Autodesk Inventor part; units mm, degrees
(part 3 of 8)
  line L1096 (-20.811, -20.7427) -> (-20.811, -20.5345) construction
  line L1097 (-20.811, -20.5345) -> (-20.6029, -20.5345) construction
  line L1098 (-20.6029, -20.5345) -> (-20.3947, -20.5345)
  spline S238 degree 2 poles (-20.3947, -20.5345) (-20.2004, -20.5345) (-20.0859, -20.4062) knots 0 0 0 1 1 1
  line L1099 (-20.3947, -20.5345) -> (-20.2004, -20.5345) construction
  line L1100 (-20.2004, -20.5345) -> (-20.0859, -20.4062) construction
  spline S239 degree 2 poles (-20.0859, -20.4062) (-19.9819, -20.2882) (-19.9819, -20.1182) knots 0 0 0 1 1 1
  line L1101 (-20.0859, -20.4062) -> (-19.9819, -20.2882) construction
  line L1102 (-19.9819, -20.2882) -> (-19.9819, -20.1182) construction
  spline S240 degree 2 poles (-19.9819, -20.1182) (-19.9819, -19.9482) (-20.0859, -19.8337) knots 0 0 0 1 1 1
  line L1103 (-19.9819, -20.1182) -> (-19.9819, -19.9482) construction
  line L1104 (-19.9819, -19.9482) -> (-20.0859, -19.8337) construction
  spline S241 degree 2 poles (-20.0859, -19.8337) (-20.2004, -19.7053) (-20.3982, -19.7053) knots 0 0 0 1 1 1
  line L1105 (-20.0859, -19.8337) -> (-20.2004, -19.7053) construction
  line L1106 (-20.2004, -19.7053) -> (-20.3982, -19.7053) construction
  line L1107 (-20.3982, -19.7053) -> (-20.6063, -19.7053)
  spline S242 degree 2 poles (-20.6063, -19.7053) (-20.8873, -19.7053) (-21.1024, -19.8719) knots 0 0 0 1 1 1
  line L1108 (-20.6063, -19.7053) -> (-20.8873, -19.7053) construction
  line L1109 (-20.8873, -19.7053) -> (-21.1024, -19.8719) construction
  spline S243 degree 2 poles (-21.1024, -19.8719) (-21.1649, -19.917) (-21.2308, -19.917) knots 0 0 0 1 1 1
  line L1110 (-21.1024, -19.8719) -> (-21.1649, -19.917) construction
  line L1111 (-21.1649, -19.917) -> (-21.2308, -19.917) construction
  spline S244 degree 2 poles (-21.2308, -19.917) (-21.3141, -19.917) (-21.439, -19.7886) (-21.439, -19.7019) knots 0 0 0 1 2 2 2
  line L1112 (-21.2308, -19.917) -> (-21.3141, -19.917) construction
  line L1113 (-21.3141, -19.917) -> (-21.439, -19.7886) construction
  line L1114 (-21.439, -19.7886) -> (-21.439, -19.7019) construction
  spline S245 degree 2 poles (-21.439, -19.7019) (-21.439, -19.6047) (-21.3522, -19.5388) knots 0 0 0 1 1 1
  line L1115 (-21.439, -19.7019) -> (-21.439, -19.6047) construction
  line L1116 (-21.439, -19.6047) -> (-21.3522, -19.5388) construction
  spline S246 degree 2 poles (-21.3522, -19.5388) (-21.0296, -19.289) (-20.6063, -19.289) knots 0 0 0 1 1 1
  line L1117 (-21.3522, -19.5388) -> (-21.0296, -19.289) construction
  line L1118 (-21.0296, -19.289) -> (-20.6063, -19.289) construction
  line L1119 (-20.6063, -19.289) -> (-20.3982, -19.289)
  spline S247 degree 2 poles (-20.3982, -19.289) (-20.0061, -19.289) (-19.7737, -19.5458) knots 0 0 0 1 1 1
  line L1120 (-20.3982, -19.289) -> (-20.0061, -19.289) construction
  line L1121 (-20.0061, -19.289) -> (-19.7737, -19.5458) construction
  spline S248 degree 2 poles (-19.7737, -19.5458) (-19.5655, -19.7817) (-19.5655, -20.1182) knots 0 0 0 1 1 1
  line L1122 (-19.7737, -19.5458) -> (-19.5655, -19.7817) construction
  line L1123 (-19.5655, -19.7817) -> (-19.5655, -20.1182) construction
  spline S249 degree 2 poles (-19.5655, -20.1182) (-19.5655, -20.5033) (-19.8257, -20.7427) knots 0 0 0 1 1 1
  line L1124 (-19.5655, -20.1182) -> (-19.5655, -20.5033) construction
  line L1125 (-19.5655, -20.5033) -> (-19.8257, -20.7427) construction
  spline S250 degree 2 poles (-19.8257, -20.7427) (-19.5655, -20.9821) (-19.5655, -21.3672) knots 0 0 0 1 1 1
  line L1126 (-19.8257, -20.7427) -> (-19.5655, -20.9821) construction
  line L1127 (-19.5655, -20.9821) -> (-19.5655, -21.3672) construction
  spline S251 degree 2 poles (-19.5655, -21.3672) (-19.5655, -21.7072) (-19.7737, -21.9396) knots 0 0 0 1 1 1
  line L1128 (-19.5655, -21.3672) -> (-19.5655, -21.7072) construction
  line L1129 (-19.5655, -21.7072) -> (-19.7737, -21.9396) construction
  spline S252 degree 2 poles (-19.7737, -21.9396) (-20.0061, -22.1963) (-20.3982, -22.1963) knots 0 0 0 1 1 1
  line L1130 (-19.7737, -21.9396) -> (-20.0061, -22.1963) construction
  line L1131 (-20.0061, -22.1963) -> (-20.3982, -22.1963) construction
  line L1132 (-20.3982, -22.1963) -> (-20.6063, -22.1963)
  spline S253 degree 2 poles (-20.6063, -22.1963) (-21.0296, -22.1963) (-21.3522, -21.9465) knots 0 0 0 1 1 1
  line L1133 (-20.6063, -22.1963) -> (-21.0296, -22.1963) construction
  line L1134 (-21.0296, -22.1963) -> (-21.3522, -21.9465) construction
  spline S254 degree 2 poles (-21.3522, -21.9465) (-21.439, -21.8806) (-21.439, -21.7835) knots 0 0 0 1 1 1
  line L1135 (-21.3522, -21.9465) -> (-21.439, -21.8806) construction
  line L1136 (-21.439, -21.8806) -> (-21.439, -21.7835) construction
  spline S255 degree 2 poles (-21.439, -21.7835) (-21.439, -21.6967) (-21.3141, -21.5684) (-21.2308, -21.5684) knots 0 0 0 1 2 2 2
  line L1137 (-21.439, -21.7835) -> (-21.439, -21.6967) construction
  line L1138 (-21.439, -21.6967) -> (-21.3141, -21.5684) construction
  line L1139 (-21.3141, -21.5684) -> (-21.2308, -21.5684) construction
  spline S256 degree 2 poles (-21.2308, -21.5684) (-21.1649, -21.5684) (-21.1024, -21.6135) knots 0 0 0 1 1 1
  line L1140 (-21.2308, -21.5684) -> (-21.1649, -21.5684) construction
  line L1141 (-21.1649, -21.5684) -> (-21.1024, -21.6135) construction
  spline S257 degree 2 poles (-21.1024, -21.6135) (-20.8873, -21.78) (-20.6063, -21.78) knots 0 0 0 1 1 1
  line L1142 (-21.1024, -21.6135) -> (-20.8873, -21.78) construction
  line L1143 (-20.8873, -21.78) -> (-20.6063, -21.78) construction
  line L1144 (-20.6063, -21.78) -> (-20.3982, -21.78)
  spline S258 degree 2 poles (-20.3982, -21.78) (-20.2004, -21.78) (-20.0859, -21.6482) knots 0 0 0 1 1 1
  line L1145 (-20.3982, -21.78) -> (-20.2004, -21.78) construction
  line L1146 (-20.2004, -21.78) -> (-20.0859, -21.6482) construction
  spline S259 degree 2 poles (-20.0859, -21.6482) (-19.9819, -21.5302) (-19.9819, -21.3602) knots 0 0 0 1 1 1
  line L1147 (-20.0859, -21.6482) -> (-19.9819, -21.5302) construction
  line L1148 (-19.9819, -21.5302) -> (-19.9819, -21.3602) construction
  spline S260 degree 2 poles (-19.9819, -21.3602) (-19.9819, -20.989) (-20.3427, -20.9508) knots 0 0 0 1 1 1
  line L1149 (-19.9819, -21.3602) -> (-19.9819, -20.989) construction
  line L1150 (-19.9819, -20.989) -> (-20.3427, -20.9508) construction
  line L1151 (-20.3427, -20.9508) -> (-20.6029, -20.9508)
  spline S261 degree 2 poles (9.298, -10.1686) (9.0898, -10.1686) (9.0898, -9.9605) knots 0 0 0 1 1 1
  line L1152 (9.298, -10.1686) -> (9.0898, -10.1686) construction
  line L1153 (9.0898, -10.1686) -> (9.0898, -9.9605) construction
  line L1154 (9.0898, -9.9605) -> (9.0898, -8.094)
  spline S262 degree 2 poles (9.0898, -8.094) (9.0898, -7.924) (8.847, -7.6777) (8.677, -7.6777) knots 0 0 0 1 2 2 2
  line L1155 (9.0898, -8.094) -> (9.0898, -7.924) construction
  line L1156 (9.0898, -7.924) -> (8.847, -7.6777) construction
  line L1157 (8.847, -7.6777) -> (8.677, -7.6777) construction
  spline S263 degree 2 poles (7.8478, -9.9605) (7.8478, -10.1686) (7.6397, -10.1686) knots 0 0 0 1 1 1
  line L1158 (7.8478, -9.9605) -> (7.8478, -10.1686) construction
  line L1159 (7.8478, -10.1686) -> (7.6397, -10.1686) construction
  spline S264 degree 2 poles (7.6397, -10.1686) (7.4315, -10.1686) (7.4315, -9.9605) knots 0 0 0 1 1 1
  line L1160 (7.6397, -10.1686) -> (7.4315, -10.1686) construction
  line L1161 (7.4315, -10.1686) -> (7.4315, -9.9605) construction
  line L1162 (7.4315, -9.9605) -> (7.4315, -7.4695)
  spline S265 degree 2 poles (7.4315, -7.4695) (7.4315, -7.2613) (7.6397, -7.2613) knots 0 0 0 1 1 1
  line L1163 (7.4315, -7.4695) -> (7.4315, -7.2613) construction
  line L1164 (7.4315, -7.2613) -> (7.6397, -7.2613) construction
  line L1165 (7.6397, -7.2613) -> (8.677, -7.2613)
  spline S266 degree 2 poles (8.677, -7.2613) (9.0204, -7.2613) (9.5062, -7.747) (9.5062, -8.0905) knots 0 0 0 1 2 2 2
  line L1166 (8.677, -7.2613) -> (9.0204, -7.2613) construction
  line L1167 (9.0204, -7.2613) -> (9.5062, -7.747) construction
  line L1168 (9.5062, -7.747) -> (9.5062, -8.0905) construction
  line L1169 (9.5062, -8.0905) -> (9.5062, -9.9605)
  spline S267 degree 2 poles (9.5062, -9.9605) (9.5062, -10.1686) (9.298, -10.1686) knots 0 0 0 1 1 1
  line L1170 (9.5062, -9.9605) -> (9.5062, -10.1686) construction
  line L1171 (9.5062, -10.1686) -> (9.298, -10.1686) construction
  spline S268 degree 2 poles (5.7697, -9.7523) (5.9397, -9.7523) (6.1825, -9.506) (6.1825, -9.336) knots 0 0 0 1 2 2 2
  line L1172 (5.7697, -9.7523) -> (5.9397, -9.7523) construction
  line L1173 (5.9397, -9.7523) -> (6.1825, -9.506) construction
  line L1174 (6.1825, -9.506) -> (6.1825, -9.336) construction
  spline S269 degree 2 poles (5.3534, -7.6777) (5.1834, -7.6777) (4.9405, -7.924) (4.9405, -8.094) knots 0 0 0 1 2 2 2
  line L1175 (5.3534, -7.6777) -> (5.1834, -7.6777) construction
  line L1176 (5.1834, -7.6777) -> (4.9405, -7.924) construction
  line L1177 (4.9405, -7.924) -> (4.9405, -8.094) construction
  line L1178 (4.9405, -8.094) -> (4.9405, -9.336)
  spline S270 degree 2 poles (4.9405, -9.336) (4.9405, -9.506) (5.1834, -9.7523) (5.3534, -9.7523) knots 0 0 0 1 2 2 2
  line L1179 (4.9405, -9.336) -> (4.9405, -9.506) construction
  line L1180 (4.9405, -9.506) -> (5.1834, -9.7523) construction
  line L1181 (5.1834, -9.7523) -> (5.3534, -9.7523) construction
  line L1182 (5.3534, -9.7523) -> (5.7697, -9.7523)
  line L1183 (5.7697, -10.1686) -> (5.3534, -10.1686)
  spline S271 degree 2 poles (5.3534, -10.1686) (5.0134, -10.1686) (4.5242, -9.6829) (4.5242, -9.3395) knots 0 0 0 1 2 2 2
  line L1184 (5.3534, -10.1686) -> (5.0134, -10.1686) construction
  line L1185 (5.0134, -10.1686) -> (4.5242, -9.6829) construction
  line L1186 (4.5242, -9.6829) -> (4.5242, -9.3395) construction
  line L1187 (4.5242, -9.3395) -> (4.5242, -8.0905)
  spline S272 degree 2 poles (4.5242, -8.0905) (4.5242, -7.747) (5.0134, -7.2613) (5.3534, -7.2613) knots 0 0 0 1 2 2 2
  line L1188 (4.5242, -8.0905) -> (4.5242, -7.747) construction
  line L1189 (4.5242, -7.747) -> (5.0134, -7.2613) construction
  line L1190 (5.0134, -7.2613) -> (5.3534, -7.2613) construction
  line L1191 (5.3534, -7.2613) -> (6.3907, -7.2613)
  spline S273 degree 2 poles (6.3907, -7.2613) (6.5989, -7.2613) (6.5989, -7.4695) knots 0 0 0 1 1 1
  line L1192 (6.3907, -7.2613) -> (6.5989, -7.2613) construction
  line L1193 (6.5989, -7.2613) -> (6.5989, -7.4695) construction
  line L1194 (6.5989, -7.4695) -> (6.5989, -9.3325)
  spline S274 degree 2 poles (6.5989, -9.3325) (6.5989, -9.6448) (6.8903, -9.7697) knots 0 0 0 1 1 1
  line L1195 (6.5989, -9.3325) -> (6.5989, -9.6448) construction
  line L1196 (6.5989, -9.6448) -> (6.8903, -9.7697) construction
  spline S275 degree 2 poles (6.8903, -9.7697) (7.0186, -9.8217) (7.0186, -9.9535) knots 0 0 0 1 1 1
  line L1197 (6.8903, -9.7697) -> (7.0186, -9.8217) construction
  line L1198 (7.0186, -9.8217) -> (7.0186, -9.9535) construction
  spline S276 degree 2 poles (7.0186, -9.9535) (7.0186, -10.0403) (6.9007, -10.1721) (6.8139, -10.1721) knots 0 0 0 1 2 2 2
  line L1199 (7.0186, -9.9535) -> (7.0186, -10.0403) construction
  line L1200 (7.0186, -10.0403) -> (6.9007, -10.1721) construction
  line L1201 (6.9007, -10.1721) -> (6.8139, -10.1721) construction
  spline S277 degree 2 poles (6.8139, -10.1721) (6.7688, -10.1721) (6.7237, -10.1513) knots 0 0 0 1 1 1
  line L1202 (6.8139, -10.1721) -> (6.7688, -10.1721) construction
  line L1203 (6.7688, -10.1721) -> (6.7237, -10.1513) construction
  spline S278 degree 2 poles (6.7237, -10.1513) (6.5156, -10.0611) (6.3872, -9.8946) knots 0 0 0 1 1 1
  line L1204 (6.7237, -10.1513) -> (6.5156, -10.0611) construction
  line L1205 (6.5156, -10.0611) -> (6.3872, -9.8946) construction
  spline S279 degree 2 poles (6.3872, -9.8946) (6.1374, -10.1686) (5.7697, -10.1686) knots 0 0 0 1 1 1
  line L1206 (6.3872, -9.8946) -> (6.1374, -10.1686) construction
  line L1207 (6.1374, -10.1686) -> (5.7697, -10.1686) construction
  spline S280 degree 2 poles (7.4738, -1.674) (7.2656, -1.674) (7.2656, -1.4659) knots 0 0 0 1 1 1
  line L1208 (7.4738, -1.674) -> (7.2656, -1.674) construction
  line L1209 (7.2656, -1.674) -> (7.2656, -1.4659) construction
  line L1210 (7.2656, -1.4659) -> (7.2656, 0.4006)
  spline S281 degree 2 poles (7.2656, 0.4006) (7.2656, 0.5706) (7.0228, 0.8169) (6.8528, 0.8169) knots 0 0 0 1 2 2 2
  line L1211 (7.2656, 0.4006) -> (7.2656, 0.5706) construction
  line L1212 (7.2656, 0.5706) -> (7.0228, 0.8169) construction
  line L1213 (7.0228, 0.8169) -> (6.8528, 0.8169) construction
  spline S282 degree 2 poles (6.0236, -1.4659) (6.0236, -1.674) (5.8155, -1.674) knots 0 0 0 1 1 1
  line L1214 (6.0236, -1.4659) -> (6.0236, -1.674) construction
  line L1215 (6.0236, -1.674) -> (5.8155, -1.674) construction
  spline S283 degree 2 poles (5.8155, -1.674) (5.6073, -1.674) (5.6073, -1.4659) knots 0 0 0 1 1 1
  line L1216 (5.8155, -1.674) -> (5.6073, -1.674) construction
  line L1217 (5.6073, -1.674) -> (5.6073, -1.4659) construction
  line L1218 (5.6073, -1.4659) -> (5.6073, 1.0251)
  spline S284 degree 2 poles (5.6073, 1.0251) (5.6073, 1.2333) (5.8155, 1.2333) knots 0 0 0 1 1 1
  line L1219 (5.6073, 1.0251) -> (5.6073, 1.2333) construction
  line L1220 (5.6073, 1.2333) -> (5.8155, 1.2333) construction
  line L1221 (5.8155, 1.2333) -> (6.8528, 1.2333)
  spline S285 degree 2 poles (6.8528, 1.2333) (7.1963, 1.2333) (7.682, 0.7475) (7.682, 0.4041) knots 0 0 0 1 2 2 2
  line L1222 (6.8528, 1.2333) -> (7.1963, 1.2333) construction
  line L1223 (7.1963, 1.2333) -> (7.682, 0.7475) construction
  line L1224 (7.682, 0.7475) -> (7.682, 0.4041) construction
  line L1225 (7.682, 0.4041) -> (7.682, -1.4659)
  spline S286 degree 2 poles (7.682, -1.4659) (7.682, -1.674) (7.4738, -1.674) knots 0 0 0 1 1 1
  line L1226 (7.682, -1.4659) -> (7.682, -1.674) construction
  line L1227 (7.682, -1.674) -> (7.4738, -1.674) construction
  spline S287 degree 2 poles (-12.3756, -9.2147) (-12.7191, -9.2147) (-13.2048, -8.729) (-13.2048, -8.3856) knots 0 0 0 1 2 2 2
  line L1228 (-12.3756, -9.2147) -> (-12.7191, -9.2147) construction
  line L1229 (-12.7191, -9.2147) -> (-13.2048, -8.729) construction
  line L1230 (-13.2048, -8.729) -> (-13.2048, -8.3856) construction
  line L1231 (-13.2048, -8.3856) -> (-13.2048, -6.9319)
  spline S288 degree 2 poles (-13.2048, -6.9319) (-13.2048, -6.7237) (-12.9966, -6.7237) knots 0 0 0 1 1 1
  line L1232 (-13.2048, -6.9319) -> (-13.2048, -6.7237) construction
  line L1233 (-13.2048, -6.7237) -> (-12.9966, -6.7237) construction
  spline S289 degree 2 poles (-12.9966, -6.7237) (-12.7885, -6.7237) (-12.7885, -6.9319) knots 0 0 0 1 1 1
  line L1234 (-12.9966, -6.7237) -> (-12.7885, -6.7237) construction
  line L1235 (-12.7885, -6.7237) -> (-12.7885, -6.9319) construction
  line L1236 (-12.7885, -6.9319) -> (-12.7885, -8.3821)
  spline S290 degree 2 poles (-12.7885, -8.3821) (-12.7885, -8.5521) (-12.5422, -8.7984) (-12.3722, -8.7984) knots 0 0 0 1 2 2 2
  line L1237 (-12.7885, -8.3821) -> (-12.7885, -8.5521) construction
  line L1238 (-12.7885, -8.5521) -> (-12.5422, -8.7984) construction
  line L1239 (-12.5422, -8.7984) -> (-12.3722, -8.7984) construction
  spline S291 degree 2 poles (-11.1301, -6.9319) (-11.1301, -6.7237) (-10.922, -6.7237) knots 0 0 0 1 1 1
  line L1240 (-11.1301, -6.9319) -> (-11.1301, -6.7237) construction
  line L1241 (-11.1301, -6.7237) -> (-10.922, -6.7237) construction
  spline S292 degree 2 poles (-10.922, -6.7237) (-10.7138, -6.7237) (-10.7138, -6.9319) knots 0 0 0 1 1 1
  line L1242 (-10.922, -6.7237) -> (-10.7138, -6.7237) construction
  line L1243 (-10.7138, -6.7237) -> (-10.7138, -6.9319) construction
  line L1244 (-10.7138, -6.9319) -> (-10.7138, -10.0474)
  spline S293 degree 2 poles (-10.7138, -10.0474) (-10.7138, -10.3908) (-11.1995, -10.8765) (-11.543, -10.8765) knots 0 0 0 1 2 2 2
  line L1245 (-10.7138, -10.0474) -> (-10.7138, -10.3908) construction
  line L1246 (-10.7138, -10.3908) -> (-11.1995, -10.8765) construction
  line L1247 (-11.1995, -10.8765) -> (-11.543, -10.8765) construction
  line L1248 (-11.543, -10.8765) -> (-12.5803, -10.8765)
  spline S294 degree 2 poles (-12.5803, -10.8765) (-12.7885, -10.8765) (-12.7885, -10.6684) knots 0 0 0 1 1 1
  line L1249 (-12.5803, -10.8765) -> (-12.7885, -10.8765) construction
  line L1250 (-12.7885, -10.8765) -> (-12.7885, -10.6684) construction
  spline S295 degree 2 poles (-12.7885, -10.6684) (-12.7885, -10.4602) (-12.5803, -10.4602) knots 0 0 0 1 1 1
  line L1251 (-12.7885, -10.6684) -> (-12.7885, -10.4602) construction
  line L1252 (-12.7885, -10.4602) -> (-12.5803, -10.4602) construction
  line L1253 (-12.5803, -10.4602) -> (-11.543, -10.4602)
  spline S296 degree 2 poles (-11.543, -10.4602) (-11.373, -10.4602) (-11.1301, -10.2139) (-11.1301, -10.0439) knots 0 0 0 1 2 2 2
  line L1254 (-11.543, -10.4602) -> (-11.373, -10.4602) construction
  line L1255 (-11.373, -10.4602) -> (-11.1301, -10.2139) construction
  line L1256 (-11.1301, -10.2139) -> (-11.1301, -10.0439) construction
  spline S297 degree 2 poles (-17.5588, -8.3856) (-17.3541, -8.3856) (-17.3541, -8.5937) knots 0 0 0 1 1 1
  line L1257 (-17.5588, -8.3856) -> (-17.3541, -8.3856) construction
  line L1258 (-17.3541, -8.3856) -> (-17.3541, -8.5937) construction
  spline S298 degree 2 poles (-17.3541, -8.5937) (-17.3541, -8.8019) (-17.5588, -8.8019) knots 0 0 0 1 1 1
  line L1259 (-17.3541, -8.5937) -> (-17.3541, -8.8019) construction
  line L1260 (-17.3541, -8.8019) -> (-17.5588, -8.8019) construction
  spline S299 degree 2 poles (-17.146, -10.4602) (-16.9378, -10.4602) (-16.9378, -10.6684) knots 0 0 0 1 1 1
  line L1261 (-17.146, -10.4602) -> (-16.9378, -10.4602) construction
  line L1262 (-16.9378, -10.4602) -> (-16.9378, -10.6684) construction
  spline S300 degree 2 poles (-16.9378, -10.6684) (-16.9378, -10.8765) (-17.146, -10.8765) knots 0 0 0 1 1 1
  line L1263 (-16.9378, -10.6684) -> (-16.9378, -10.8765) construction
  line L1264 (-16.9378, -10.8765) -> (-17.146, -10.8765) construction
  line L1265 (-17.146, -10.8765) -> (-18.8112, -10.8765)
  spline S301 degree 2 poles (-18.8112, -10.8765) (-19.0194, -10.8765) (-19.0194, -10.6823) knots 0 0 0 1 1 1
  line L1266 (-18.8112, -10.8765) -> (-19.0194, -10.8765) construction
  line L1267 (-19.0194, -10.8765) -> (-19.0194, -10.6823) construction
  line L1268 (-19.0194, -10.6823) -> (-19.0194, -6.9319)
  spline S302 degree 2 poles (-19.0194, -6.9319) (-19.0194, -6.7237) (-18.8112, -6.7237) knots 0 0 0 1 1 1
  line L1269 (-19.0194, -6.9319) -> (-19.0194, -6.7237) construction
  line L1270 (-19.0194, -6.7237) -> (-18.8112, -6.7237) construction
  line L1271 (-18.8112, -6.7237) -> (-17.146, -6.7237)
  spline S303 degree 2 poles (-17.146, -6.7237) (-16.9378, -6.7237) (-16.9378, -6.9319) knots 0 0 0 1 1 1
  line L1272 (-17.146, -6.7237) -> (-16.9378, -6.7237) construction
  line L1273 (-16.9378, -6.7237) -> (-16.9378, -6.9319) construction
  spline S304 degree 2 poles (-16.9378, -6.9319) (-16.9378, -7.1401) (-17.146, -7.1401) knots 0 0 0 1 1 1
  line L1274 (-16.9378, -6.9319) -> (-16.9378, -7.1401) construction
  line L1275 (-16.9378, -7.1401) -> (-17.146, -7.1401) construction
  spline S305 degree 2 poles (-17.2667, 3.6542) (-17.7004, 3.6542) (-18.3075, 4.2614) (-18.3075, 4.6916) knots 0 0 0 1 2 2 2
  line L1276 (-17.2667, 3.6542) -> (-17.7004, 3.6542) construction
  line L1277 (-17.7004, 3.6542) -> (-18.3075, 4.2614) construction
  line L1278 (-18.3075, 4.2614) -> (-18.3075, 4.6916) construction
  line L1279 (-18.3075, 4.6916) -> (-18.3075, 6.7697)
  spline S306 degree 2 poles (-18.3075, 6.7697) (-18.3075, 7.1964) (-17.7004, 7.807) (-17.2667, 7.807) knots 0 0 0 1 2 2 2
  line L1280 (-18.3075, 6.7697) -> (-18.3075, 7.1964) construction
  line L1281 (-18.3075, 7.1964) -> (-17.7004, 7.807) construction
  line L1282 (-17.7004, 7.807) -> (-17.2667, 7.807) construction
  line L1283 (-17.2667, 7.807) -> (-16.4376, 7.807)
  spline S307 degree 2 poles (-16.4376, 7.807) (-16.2294, 7.807) (-16.2294, 7.5989) knots 0 0 0 1 1 1
  line L1284 (-16.4376, 7.807) -> (-16.2294, 7.807) construction
  line L1285 (-16.2294, 7.807) -> (-16.2294, 7.5989) construction
  spline S308 degree 2 poles (-16.2294, 7.5989) (-16.2294, 7.3907) (-16.4376, 7.3907) knots 0 0 0 1 1 1
  line L1286 (-16.2294, 7.5989) -> (-16.2294, 7.3907) construction
  line L1287 (-16.2294, 7.3907) -> (-16.4376, 7.3907) construction
  line L1288 (-16.4376, 7.3907) -> (-17.2667, 7.3907)
  spline S309 degree 2 poles (-17.2667, 7.3907) (-17.5269, 7.3907) (-17.8912, 7.0264) (-17.8912, 6.7697) knots 0 0 0 1 2 2 2
  line L1289 (-17.2667, 7.3907) -> (-17.5269, 7.3907) construction
  line L1290 (-17.5269, 7.3907) -> (-17.8912, 7.0264) construction
  line L1291 (-17.8912, 7.0264) -> (-17.8912, 6.7697) construction
  line L1292 (-17.8912, 6.7697) -> (-17.8912, 4.6916)
  spline S310 degree 2 poles (-17.8912, 4.6916) (-17.8912, 4.4348) (-17.5269, 4.0705) (-17.2667, 4.0705) knots 0 0 0 1 2 2 2
  line L1293 (-17.8912, 4.6916) -> (-17.8912, 4.4348) construction
  line L1294 (-17.8912, 4.4348) -> (-17.5269, 4.0705) construction
  line L1295 (-17.5269, 4.0705) -> (-17.2667, 4.0705) construction
  line L1296 (-17.2667, 4.0705) -> (-16.4376, 4.0705)
  spline S311 degree 2 poles (-16.4376, 4.0705) (-16.2294, 4.0705) (-16.2294, 3.8624) knots 0 0 0 1 1 1
  line L1297 (-16.4376, 4.0705) -> (-16.2294, 4.0705) construction
  line L1298 (-16.2294, 4.0705) -> (-16.2294, 3.8624) construction
  spline S312 degree 2 poles (-16.2294, 3.8624) (-16.2294, 3.6542) (-16.4376, 3.6542) knots 0 0 0 1 1 1
  line L1299 (-16.2294, 3.8624) -> (-16.2294, 3.6542) construction
  line L1300 (-16.2294, 3.6542) -> (-16.4376, 3.6542) construction
  line L1301 (-16.4376, 3.6542) -> (-17.2667, 3.6542)
  spline S313 degree 2 poles (-8.8573, -1.3741) (-8.6873, -1.3741) (-8.4445, -1.1278) (-8.4445, -0.9578) knots 0 0 0 1 2 2 2
  line L1302 (-8.8573, -1.3741) -> (-8.6873, -1.3741) construction
  line L1303 (-8.6873, -1.3741) -> (-8.4445, -1.1278) construction
  line L1304 (-8.4445, -1.1278) -> (-8.4445, -0.9578) construction
  line L1305 (-8.4445, -0.9578) -> (-8.4445, 0.2842)
  spline S314 degree 2 poles (-8.4445, 0.2842) (-8.4445, 0.4542) (-8.6873, 0.7006) (-8.8573, 0.7006) knots 0 0 0 1 2 2 2
  line L1306 (-8.4445, 0.2842) -> (-8.4445, 0.4542) construction
  line L1307 (-8.4445, 0.4542) -> (-8.6873, 0.7006) construction
  line L1308 (-8.6873, 0.7006) -> (-8.8573, 0.7006) construction
  spline S315 degree 2 poles (-9.6865, -2.8277) (-9.6865, -3.0359) (-9.8947, -3.0359) knots 0 0 0 1 1 1
  line L1309 (-9.6865, -2.8277) -> (-9.6865, -3.0359) construction
  line L1310 (-9.6865, -3.0359) -> (-9.8947, -3.0359) construction
  spline S316 degree 2 poles (-9.8947, -3.0359) (-10.1028, -3.0359) (-10.1028, -2.8277) knots 0 0 0 1 1 1
  line L1311 (-9.8947, -3.0359) -> (-10.1028, -3.0359) construction
  line L1312 (-10.1028, -3.0359) -> (-10.1028, -2.8277) construction
  line L1313 (-10.1028, -2.8277) -> (-10.1028, 0.9087)
  spline S317 degree 2 poles (-10.1028, 0.9087) (-10.1028, 1.1169) (-9.8947, 1.1169) knots 0 0 0 1 1 1
  line L1314 (-10.1028, 0.9087) -> (-10.1028, 1.1169) construction
  line L1315 (-10.1028, 1.1169) -> (-9.8947, 1.1169) construction
  line L1316 (-9.8947, 1.1169) -> (-8.8573, 1.1169)
  spline S318 degree 2 poles (-8.8573, 1.1169) (-8.5139, 1.1169) (-8.0282, 0.6312) (-8.0282, 0.2877) knots 0 0 0 1 2 2 2
  line L1317 (-8.8573, 1.1169) -> (-8.5139, 1.1169) construction
  line L1318 (-8.5139, 1.1169) -> (-8.0282, 0.6312) construction
  line L1319 (-8.0282, 0.6312) -> (-8.0282, 0.2877) construction
  line L1320 (-8.0282, 0.2877) -> (-8.0282, -0.9612)
  spline S319 degree 2 poles (-8.0282, -0.9612) (-8.0282, -1.3047) (-8.5139, -1.7904) (-8.8573, -1.7904) knots 0 0 0 1 2 2 2
  line L1321 (-8.0282, -0.9612) -> (-8.0282, -1.3047) construction
  line L1322 (-8.0282, -1.3047) -> (-8.5139, -1.7904) construction
  line L1323 (-8.5139, -1.7904) -> (-8.8573, -1.7904) construction
  spline S320 degree 2 poles (-17.1664, 0.9087) (-17.1664, 1.1169) (-16.9582, 1.1169) knots 0 0 0 1 1 1
  line L1324 (-17.1664, 0.9087) -> (-17.1664, 1.1169) construction
  line L1325 (-17.1664, 1.1169) -> (-16.9582, 1.1169) construction
  spline S321 degree 2 poles (-16.9582, 1.1169) (-16.7501, 1.1169) (-16.7501, 0.9087) knots 0 0 0 1 1 1
  line L1326 (-16.9582, 1.1169) -> (-16.7501, 1.1169) construction
  line L1327 (-16.7501, 1.1169) -> (-16.7501, 0.9087) construction
  line L1328 (-16.7501, 0.9087) -> (-16.7501, -1.5823)
  spline S322 degree 2 poles (-16.7501, -1.5823) (-16.7501, -1.7904) (-16.9582, -1.7904) knots 0 0 0 1 1 1
  line L1329 (-16.7501, -1.5823) -> (-16.7501, -1.7904) construction
  line L1330 (-16.7501, -1.7904) -> (-16.9582, -1.7904) construction
  spline S323 degree 2 poles (-16.9582, -1.7904) (-17.1664, -1.7904) (-17.1664, -1.5823) knots 0 0 0 1 1 1
  line L1331 (-16.9582, -1.7904) -> (-17.1664, -1.7904) construction
  line L1332 (-17.1664, -1.7904) -> (-17.1664, -1.5823) construction
  spline S324 degree 2 poles (-18.4084, -1.5823) (-18.4084, -1.7904) (-18.6166, -1.7904) knots 0 0 0 1 1 1
  line L1333 (-18.4084, -1.5823) -> (-18.4084, -1.7904) construction
  line L1334 (-18.4084, -1.7904) -> (-18.6166, -1.7904) construction
  spline S325 degree 2 poles (-18.6166, -1.7904) (-18.8247, -1.7904) (-18.8247, -1.5823) knots 0 0 0 1 1 1
  line L1335 (-18.6166, -1.7904) -> (-18.8247, -1.7904) construction
  line L1336 (-18.8247, -1.7904) -> (-18.8247, -1.5823) construction
  line L1337 (-18.8247, -1.5823) -> (-18.8247, 0.9087)
  spline S326 degree 2 poles (-18.8247, 0.9087) (-18.8247, 1.1169) (-18.6166, 1.1169) knots 0 0 0 1 1 1
  line L1338 (-18.8247, 0.9087) -> (-18.8247, 1.1169) construction
  line L1339 (-18.8247, 1.1169) -> (-18.6166, 1.1169) construction
  spline S327 degree 2 poles (-18.6166, 1.1169) (-18.4084, 1.1169) (-18.4084, 0.9087) knots 0 0 0 1 1 1
  line L1340 (-18.6166, 1.1169) -> (-18.4084, 1.1169) construction
  line L1341 (-18.4084, 1.1169) -> (-18.4084, 0.9087) construction
  spline S328 degree 2 poles (16.7676, 22.7837) (16.7676, 22.5747) (16.5586, 22.5747) knots 0 0 0 1 1 1
  line L1342 (16.7676, 22.7837) -> (16.7676, 22.5747) construction
  line L1343 (16.7676, 22.5747) -> (16.5586, 22.5747) construction
  spline S329 degree 2 poles (16.5586, 22.5747) (16.3496, 22.5747) (16.3496, 22.7837) knots 0 0 0 1 1 1
  line L1344 (16.5586, 22.5747) -> (16.3496, 22.5747) construction
  line L1345 (16.3496, 22.5747) -> (16.3496, 22.7837) construction
  line L1346 (16.3496, 22.7837) -> (16.3496, 24.7199)
  spline S330 degree 2 poles (16.3496, 24.7199) (16.3496, 24.9289) (16.5586, 24.9289) knots 0 0 0 1 1 1
  line L1347 (16.3496, 24.7199) -> (16.3496, 24.9289) construction
  line L1348 (16.3496, 24.9289) -> (16.5586, 24.9289) construction
  line L1349 (16.5586, 24.9289) -> (18.008, 24.9289)
  spline S331 degree 2 poles (18.008, 24.9289) (18.2968, 24.9289) (18.7038, 24.5219) (18.7038, 24.2359) knots 0 0 0 1 2 2 2
  line L1350 (18.008, 24.9289) -> (18.2968, 24.9289) construction
  line L1351 (18.2968, 24.9289) -> (18.7038, 24.5219) construction
  line L1352 (18.7038, 24.5219) -> (18.7038, 24.2359) construction
  line L1353 (18.7038, 24.2359) -> (18.7038, 22.7837)
  spline S332 degree 2 poles (18.7038, 22.7837) (18.7038, 22.5747) (18.4948, 22.5747) knots 0 0 0 1 1 1
  line L1354 (18.7038, 22.7837) -> (18.7038, 22.5747) construction
  line L1355 (18.7038, 22.5747) -> (18.4948, 22.5747) construction
  spline S333 degree 2 poles (18.4948, 22.5747) (18.2858, 22.5747) (18.2858, 22.7837) knots 0 0 0 1 1 1
  line L1356 (18.4948, 22.5747) -> (18.2858, 22.5747) construction
  line L1357 (18.2858, 22.5747) -> (18.2858, 22.7837) construction
  line L1358 (18.2858, 22.7837) -> (18.2858, 24.2386)
  spline S334 degree 2 poles (18.2858, 24.2386) (18.2858, 24.3486) (18.1208, 24.5136) (18.0107, 24.5136) knots 0 0 0 1 2 2 2
  line L1359 (18.2858, 24.2386) -> (18.2858, 24.3486) construction
  line L1360 (18.2858, 24.3486) -> (18.1208, 24.5136) construction
  line L1361 (18.1208, 24.5136) -> (18.0107, 24.5136) construction
  spline S335 degree 2 poles (17.7357, 22.7837) (17.7357, 22.5747) (17.5267, 22.5747) knots 0 0 0 1 1 1
  line L1362 (17.7357, 22.7837) -> (17.7357, 22.5747) construction
  line L1363 (17.7357, 22.5747) -> (17.5267, 22.5747) construction
  spline S336 degree 2 poles (17.5267, 22.5747) (17.3177, 22.5747) (17.3177, 22.7837) knots 0 0 0 1 1 1
  line L1364 (17.5267, 22.5747) -> (17.3177, 22.5747) construction
  line L1365 (17.3177, 22.5747) -> (17.3177, 22.7837) construction
  spline S337 degree 2 poles (13.327, 22.5747) (13.118, 22.5747) (13.118, 22.7837) knots 0 0 0 1 1 1
  line L1366 (13.327, 22.5747) -> (13.118, 22.5747) construction
  line L1367 (13.118, 22.5747) -> (13.118, 22.7837) construction
  line L1368 (13.118, 22.7837) -> (13.118, 24.2386)
  spline S338 degree 2 poles (13.118, 24.2386) (13.118, 24.3486) (12.953, 24.5136) (12.8402, 24.5136) knots 0 0 0 1 2 2 2
  line L1369 (13.118, 24.2386) -> (13.118, 24.3486) construction
  line L1370 (13.118, 24.3486) -> (12.953, 24.5136) construction
  line L1371 (12.953, 24.5136) -> (12.8402, 24.5136) construction
  spline S339 degree 2 poles (12.2407, 22.7837) (12.2407, 22.5747) (12.0317, 22.5747) knots 0 0 0 1 1 1
  line L1372 (12.2407, 22.7837) -> (12.2407, 22.5747) construction
  line L1373 (12.2407, 22.5747) -> (12.0317, 22.5747) construction
  spline S340 degree 2 poles (12.0317, 22.5747) (11.8226, 22.5747) (11.8226, 22.7837) knots 0 0 0 1 1 1
  line L1374 (12.0317, 22.5747) -> (11.8226, 22.5747) construction
  line L1375 (11.8226, 22.5747) -> (11.8226, 22.7837) construction
  line L1376 (11.8226, 22.7837) -> (11.8226, 24.7199)
  spline S341 degree 2 poles (11.8226, 24.7199) (11.8226, 24.9289) (12.0317, 24.9289) knots 0 0 0 1 1 1
  line L1377 (11.8226, 24.7199) -> (11.8226, 24.9289) construction
  line L1378 (11.8226, 24.9289) -> (12.0317, 24.9289) construction
  line L1379 (12.0317, 24.9289) -> (12.8402, 24.9289)
  spline S342 degree 2 poles (12.8402, 24.9289) (13.129, 24.9289) (13.5361, 24.5219) (13.5361, 24.2359) knots 0 0 0 1 2 2 2
  line L1380 (12.8402, 24.9289) -> (13.129, 24.9289) construction
  line L1381 (13.129, 24.9289) -> (13.5361, 24.5219) construction
  line L1382 (13.5361, 24.5219) -> (13.5361, 24.2359) construction
  line L1383 (13.5361, 24.2359) -> (13.5361, 22.7837)
  spline S343 degree 2 poles (13.5361, 22.7837) (13.5361, 22.5747) (13.327, 22.5747) knots 0 0 0 1 1 1
  line L1384 (13.5361, 22.7837) -> (13.5361, 22.5747) construction
  line L1385 (13.5361, 22.5747) -> (13.327, 22.5747) construction
  spline S344 degree 2 poles (-7.3596, 13.1349) (-7.5678, 13.1349) (-7.5678, 13.3431) knots 0 0 0 1 1 1
  line L1386 (-7.3596, 13.1349) -> (-7.5678, 13.1349) construction
  line L1387 (-7.5678, 13.1349) -> (-7.5678, 13.3431) construction
  spline S345 degree 2 poles (-8.4247, 14.873) (-8.5045, 14.7412) (-8.6051, 14.7412) knots 0 0 0 1 1 1
  line L1388 (-8.4247, 14.873) -> (-8.5045, 14.7412) construction
  line L1389 (-8.5045, 14.7412) -> (-8.6051, 14.7412) construction
  spline S346 degree 2 poles (-8.6051, 14.7412) (-8.7057, 14.7412) (-8.782, 14.873) knots 0 0 0 1 1 1
  line L1390 (-8.6051, 14.7412) -> (-8.7057, 14.7412) construction
  line L1391 (-8.7057, 14.7412) -> (-8.782, 14.873) construction
  spline S347 degree 2 poles (-9.6459, 13.3431) (-9.6459, 13.1349) (-9.8541, 13.1349) knots 0 0 0 1 1 1
  line L1392 (-9.6459, 13.3431) -> (-9.6459, 13.1349) construction
  line L1393 (-9.6459, 13.1349) -> (-9.8541, 13.1349) construction
  spline S348 degree 2 poles (-9.8541, 13.1349) (-10.0622, 13.1349) (-10.0622, 13.3431) knots 0 0 0 1 1 1
  line L1394 (-9.8541, 13.1349) -> (-10.0622, 13.1349) construction
  line L1395 (-10.0622, 13.1349) -> (-10.0622, 13.3431) construction
  line L1396 (-10.0622, 13.3431) -> (-10.0622, 17.0622)
  spline S349 degree 2 poles (-10.0622, 17.0622) (-10.0622, 17.3016) (-9.8749, 17.3016) knots 0 0 0 1 1 1
  line L1397 (-10.0622, 17.0622) -> (-10.0622, 17.3016) construction
  line L1398 (-10.0622, 17.3016) -> (-9.8749, 17.3016) construction
  spline S350 degree 2 poles (-9.8749, 17.3016) (-9.7534, 17.3016) (-9.6737, 17.1697) knots 0 0 0 1 1 1
  line L1399 (-9.8749, 17.3016) -> (-9.7534, 17.3016) construction
  line L1400 (-9.7534, 17.3016) -> (-9.6737, 17.1697) construction
  spline S351 degree 2 poles (-7.54, 17.1697) (-7.4602, 17.3016) (-7.3423, 17.3016) knots 0 0 0 1 1 1
  line L1401 (-7.54, 17.1697) -> (-7.4602, 17.3016) construction
  line L1402 (-7.4602, 17.3016) -> (-7.3423, 17.3016) construction
  spline S352 degree 2 poles (-7.3423, 17.3016) (-7.1514, 17.3016) (-7.1514, 17.0622) knots 0 0 0 1 1 1
  line L1403 (-7.3423, 17.3016) -> (-7.1514, 17.3016) construction
  line L1404 (-7.1514, 17.3016) -> (-7.1514, 17.0622) construction
  line L1405 (-7.1514, 17.0622) -> (-7.1514, 13.3431)
  spline S353 degree 2 poles (-7.1514, 13.3431) (-7.1514, 13.1349) (-7.3596, 13.1349) knots 0 0 0 1 1 1
  line L1406 (-7.1514, 13.3431) -> (-7.1514, 13.1349) construction
  line L1407 (-7.1514, 13.1349) -> (-7.3596, 13.1349) construction
  line L1408 (-14.4266, 13.1349) -> (-15.6721, 13.1349)
  spline S354 degree 2 poles (-15.6721, 13.1349) (-16.1023, 13.1349) (-16.7095, 13.742) (-16.7095, 14.1722) knots 0 0 0 1 2 2 2
  line L1409 (-15.6721, 13.1349) -> (-16.1023, 13.1349) construction
  line L1410 (-16.1023, 13.1349) -> (-16.7095, 13.742) construction
  line L1411 (-16.7095, 13.742) -> (-16.7095, 14.1722) construction
  line L1412 (-16.7095, 14.1722) -> (-16.7095, 16.2504)
  spline S355 degree 2 poles (-16.7095, 16.2504) (-16.7095, 16.6806) (-16.1023, 17.2877) (-15.6721, 17.2877) knots 0 0 0 1 2 2 2
  line L1413 (-16.7095, 16.2504) -> (-16.7095, 16.6806) construction
  line L1414 (-16.7095, 16.6806) -> (-16.1023, 17.2877) construction
  line L1415 (-16.1023, 17.2877) -> (-15.6721, 17.2877) construction
  line L1416 (-15.6721, 17.2877) -> (-14.4266, 17.2877)
  spline S356 degree 2 poles (-14.4266, 17.2877) (-14.2185, 17.2877) (-14.2185, 17.0795) knots 0 0 0 1 1 1
  line L1417 (-14.4266, 17.2877) -> (-14.2185, 17.2877) construction
  line L1418 (-14.2185, 17.2877) -> (-14.2185, 17.0795) construction
  spline S357 degree 2 poles (-14.2185, 17.0795) (-14.2185, 16.8714) (-14.4266, 16.8714) knots 0 0 0 1 1 1
  line L1419 (-14.2185, 17.0795) -> (-14.2185, 16.8714) construction
  line L1420 (-14.2185, 16.8714) -> (-14.4266, 16.8714) construction
  line L1421 (-14.4266, 16.8714) -> (-15.6721, 16.8714)
  spline S358 degree 2 poles (-15.6721, 16.8714) (-15.9289, 16.8714) (-16.2931, 16.5071) (-16.2931, 16.2504) knots 0 0 0 1 2 2 2
  line L1422 (-15.6721, 16.8714) -> (-15.9289, 16.8714) construction
  line L1423 (-15.9289, 16.8714) -> (-16.2931, 16.5071) construction
  line L1424 (-16.2931, 16.5071) -> (-16.2931, 16.2504) construction
  line L1425 (-16.2931, 16.2504) -> (-16.2931, 14.1722)
  spline S359 degree 2 poles (-16.2931, 14.1722) (-16.2931, 13.9155) (-15.9289, 13.5512) (-15.6721, 13.5512) knots 0 0 0 1 2 2 2
  line L1426 (-16.2931, 14.1722) -> (-16.2931, 13.9155) construction
  line L1427 (-16.2931, 13.9155) -> (-15.9289, 13.5512) construction
  line L1428 (-15.9289, 13.5512) -> (-15.6721, 13.5512) construction
  spline S360 degree 2 poles (-14.8395, 15.2096) (-15.0476, 15.2096) (-15.0476, 15.4177) knots 0 0 0 1 1 1
  line L1429 (-14.8395, 15.2096) -> (-15.0476, 15.2096) construction
  line L1430 (-15.0476, 15.2096) -> (-15.0476, 15.4177) construction
  spline S361 degree 2 poles (-15.0476, 15.4177) (-15.0476, 15.6259) (-14.8395, 15.6259) knots 0 0 0 1 1 1
  line L1431 (-15.0476, 15.4177) -> (-15.0476, 15.6259) construction
  line L1432 (-15.0476, 15.6259) -> (-14.8395, 15.6259) construction
  line L1433 (-14.8395, 15.6259) -> (-14.4266, 15.6259)
  spline S362 degree 2 poles (-14.4266, 15.6259) (-14.3434, 15.6259) (-14.2185, 15.501) (-14.2185, 15.4177) knots 0 0 0 1 2 2 2
  line L1434 (-14.4266, 15.6259) -> (-14.3434, 15.6259) construction
  line L1435 (-14.3434, 15.6259) -> (-14.2185, 15.501) construction
  line L1436 (-14.2185, 15.501) -> (-14.2185, 15.4177) construction
  line L1437 (-14.2185, 15.4177) -> (-14.2185, 13.3431)
  spline S363 degree 2 poles (-14.2185, 13.3431) (-14.2185, 13.2598) (-14.3434, 13.1349) (-14.4266, 13.1349) knots 0 0 0 1 2 2 2
  line L1438 (-14.2185, 13.3431) -> (-14.2185, 13.2598) construction
  line L1439 (-14.2185, 13.2598) -> (-14.3434, 13.1349) construction
  line L1440 (-14.3434, 13.1349) -> (-14.4266, 13.1349) construction
  line L1441 (-14.4134, 18.1752) -> (-15.6588, 18.1752)
  spline S364 degree 2 poles (-15.6588, 18.1752) (-16.089, 18.1752) (-16.6962, 18.7824) (-16.6962, 19.2126) knots 0 0 0 1 2 2 2
  line L1442 (-15.6588, 18.1752) -> (-16.089, 18.1752) construction
  line L1443 (-16.089, 18.1752) -> (-16.6962, 18.7824) construction
  line L1444 (-16.6962, 18.7824) -> (-16.6962, 19.2126) construction
  line L1445 (-16.6962, 19.2126) -> (-16.6962, 21.2907)
  spline S365 degree 2 poles (-16.6962, 21.2907) (-16.6962, 21.7209) (-16.089, 22.328) (-15.6588, 22.328) knots 0 0 0 1 2 2 2
  line L1446 (-16.6962, 21.2907) -> (-16.6962, 21.7209) construction
  line L1447 (-16.6962, 21.7209) -> (-16.089, 22.328) construction
  line L1448 (-16.089, 22.328) -> (-15.6588, 22.328) construction
  line L1449 (-15.6588, 22.328) -> (-14.4134, 22.328)
  spline S366 degree 2 poles (-14.4134, 22.328) (-14.2052, 22.328) (-14.2052, 22.1199) knots 0 0 0 1 1 1
  line L1450 (-14.4134, 22.328) -> (-14.2052, 22.328) construction
  line L1451 (-14.2052, 22.328) -> (-14.2052, 22.1199) construction
  spline S367 degree 2 poles (-14.2052, 22.1199) (-14.2052, 21.9117) (-14.4134, 21.9117) knots 0 0 0 1 1 1
  line L1452 (-14.2052, 22.1199) -> (-14.2052, 21.9117) construction
  line L1453 (-14.2052, 21.9117) -> (-14.4134, 21.9117) construction
  line L1454 (-14.4134, 21.9117) -> (-15.6588, 21.9117)
  spline S368 degree 2 poles (-15.6588, 21.9117) (-15.9156, 21.9117) (-16.2799, 21.5474) (-16.2799, 21.2907) knots 0 0 0 1 2 2 2
  line L1455 (-15.6588, 21.9117) -> (-15.9156, 21.9117) construction
  line L1456 (-15.9156, 21.9117) -> (-16.2799, 21.5474) construction
  line L1457 (-16.2799, 21.5474) -> (-16.2799, 21.2907) construction
  line L1458 (-16.2799, 21.2907) -> (-16.2799, 19.2126)
  spline S369 degree 2 poles (-16.2799, 19.2126) (-16.2799, 18.9558) (-15.9156, 18.5916) (-15.6588, 18.5916) knots 0 0 0 1 2 2 2
  line L1459 (-16.2799, 19.2126) -> (-16.2799, 18.9558) construction
  line L1460 (-16.2799, 18.9558) -> (-15.9156, 18.5916) construction
  line L1461 (-15.9156, 18.5916) -> (-15.6588, 18.5916) construction
  spline S370 degree 2 poles (-14.8262, 20.2499) (-15.0344, 20.2499) (-15.0344, 20.4581) knots 0 0 0 1 1 1
  line L1462 (-14.8262, 20.2499) -> (-15.0344, 20.2499) construction
  line L1463 (-15.0344, 20.2499) -> (-15.0344, 20.4581) construction
  spline S371 degree 2 poles (-15.0344, 20.4581) (-15.0344, 20.6662) (-14.8262, 20.6662) knots 0 0 0 1 1 1
  line L1464 (-15.0344, 20.4581) -> (-15.0344, 20.6662) construction
  line L1465 (-15.0344, 20.6662) -> (-14.8262, 20.6662) construction
  line L1466 (-14.8262, 20.6662) -> (-14.4134, 20.6662)
  spline S372 degree 2 poles (-14.4134, 20.6662) (-14.3301, 20.6662) (-14.2052, 20.5413) (-14.2052, 20.4581) knots 0 0 0 1 2 2 2
  line L1467 (-14.4134, 20.6662) -> (-14.3301, 20.6662) construction
  line L1468 (-14.3301, 20.6662) -> (-14.2052, 20.5413) construction
  line L1469 (-14.2052, 20.5413) -> (-14.2052, 20.4581) construction
  line L1470 (-14.2052, 20.4581) -> (-14.2052, 18.3834)
  spline S373 degree 2 poles (-14.2052, 18.3834) (-14.2052, 18.3001) (-14.3301, 18.1752) (-14.4134, 18.1752) knots 0 0 0 1 2 2 2
  line L1471 (-14.2052, 18.3834) -> (-14.2052, 18.3001) construction
  line L1472 (-14.2052, 18.3001) -> (-14.3301, 18.1752) construction
  line L1473 (-14.3301, 18.1752) -> (-14.4134, 18.1752) construction
  spline S374 degree 2 poles (-9.7269, 30.0012) (-10.2559, 30.0012) (-10.9966, 30.7419) (-10.9966, 31.2667) knots 0 0 0 1 2 2 2
  line L1474 (-9.7269, 30.0012) -> (-10.2559, 30.0012) construction
  line L1475 (-10.2559, 30.0012) -> (-10.9966, 30.7419) construction
  line L1476 (-10.9966, 30.7419) -> (-10.9966, 31.2667) construction
  line L1477 (-10.9966, 31.2667) -> (-10.9966, 33.802)
  spline S375 degree 2 poles (-10.9966, 33.802) (-10.9966, 34.3227) (-10.2559, 35.0676) (-9.7269, 35.0676) knots 0 0 0 1 2 2 2
  line L1478 (-10.9966, 33.802) -> (-10.9966, 34.3227) construction
  line L1479 (-10.9966, 34.3227) -> (-10.2559, 35.0676) construction
  line L1480 (-10.2559, 35.0676) -> (-9.7269, 35.0676) construction
  line L1481 (-9.7269, 35.0676) -> (-8.7153, 35.0676)
  spline S376 degree 2 poles (-8.7153, 35.0676) (-8.4613, 35.0676) (-8.4613, 34.8136) knots 0 0 0 1 1 1
  line L1482 (-8.7153, 35.0676) -> (-8.4613, 35.0676) construction
  line L1483 (-8.4613, 35.0676) -> (-8.4613, 34.8136) construction
  spline S377 degree 2 poles (-8.4613, 34.8136) (-8.4613, 34.5597) (-8.7153, 34.5597) knots 0 0 0 1 1 1
  line L1484 (-8.4613, 34.8136) -> (-8.4613, 34.5597) construction
  line L1485 (-8.4613, 34.5597) -> (-8.7153, 34.5597) construction
  line L1486 (-8.7153, 34.5597) -> (-9.7269, 34.5597)
  spline S378 degree 2 poles (-9.7269, 34.5597) (-10.0443, 34.5597) (-10.4887, 34.1153) (-10.4887, 33.802) knots 0 0 0 1 2 2 2
  line L1487 (-9.7269, 34.5597) -> (-10.0443, 34.5597) construction
  line L1488 (-10.0443, 34.5597) -> (-10.4887, 34.1153) construction
  line L1489 (-10.4887, 34.1153) -> (-10.4887, 33.802) construction
  line L1490 (-10.4887, 33.802) -> (-10.4887, 31.2667)
  spline S379 degree 2 poles (-10.4887, 31.2667) (-10.4887, 30.9535) (-10.0443, 30.5091) (-9.7269, 30.5091) knots 0 0 0 1 2 2 2
  line L1491 (-10.4887, 31.2667) -> (-10.4887, 30.9535) construction
  line L1492 (-10.4887, 30.9535) -> (-10.0443, 30.5091) construction
  line L1493 (-10.0443, 30.5091) -> (-9.7269, 30.5091) construction
  line L1494 (-9.7269, 30.5091) -> (-8.7153, 30.5091)
  spline S380 degree 2 poles (-8.7153, 30.5091) (-8.4613, 30.5091) (-8.4613, 30.2551) knots 0 0 0 1 1 1
  line L1495 (-8.7153, 30.5091) -> (-8.4613, 30.5091) construction
  line L1496 (-8.4613, 30.5091) -> (-8.4613, 30.2551) construction
  spline S381 degree 2 poles (-8.4613, 30.2551) (-8.4613, 30.0012) (-8.7153, 30.0012) knots 0 0 0 1 1 1
  line L1497 (-8.4613, 30.2551) -> (-8.4613, 30.0012) construction
  line L1498 (-8.4613, 30.0012) -> (-8.7153, 30.0012) construction
  line L1499 (-8.7153, 30.0012) -> (-9.7269, 30.0012)
  spline S382 degree 2 poles (-15.0388, 30.179) (-15.0938, 30.0054) (-15.2673, 30.0054) knots 0 0 0 1 1 1
  line L1500 (-15.0388, 30.179) -> (-15.0938, 30.0054) construction
  line L1501 (-15.0938, 30.0054) -> (-15.2673, 30.0054) construction
  spline S383 degree 2 poles (-15.2673, 30.0054) (-15.5297, 30.0054) (-15.5297, 30.2467) knots 0 0 0 1 1 1
  line L1502 (-15.2673, 30.0054) -> (-15.5297, 30.0054) construction
  line L1503 (-15.5297, 30.0054) -> (-15.5297, 30.2467) construction
  spline S384 degree 2 poles (-15.5297, 30.2467) (-15.5297, 30.2932) (-15.5128, 30.3398) knots 0 0 0 1 1 1
  line L1504 (-15.5297, 30.2467) -> (-15.5297, 30.2932) construction
  line L1505 (-15.5297, 30.2932) -> (-15.5128, 30.3398) construction
  line L1506 (-15.5128, 30.3398) -> (-13.9891, 34.9025)
  spline S385 degree 2 poles (-13.9891, 34.9025) (-13.9171, 35.1184) (-13.7521, 35.1184) knots 0 0 0 1 1 1
  line L1507 (-13.9891, 34.9025) -> (-13.9171, 35.1184) construction
  line L1508 (-13.9171, 35.1184) -> (-13.7521, 35.1184) construction
  spline S386 degree 2 poles (-13.7521, 35.1184) (-13.5828, 35.1184) (-13.515, 34.9025) knots 0 0 0 1 1 1
  line L1509 (-13.7521, 35.1184) -> (-13.5828, 35.1184) construction
  line L1510 (-13.5828, 35.1184) -> (-13.515, 34.9025) construction
  line L1511 (-13.515, 34.9025) -> (-11.9913, 30.3398)
  spline S387 degree 2 poles (-11.9913, 30.3398) (-11.9786, 30.2932) (-11.9786, 30.2467) knots 0 0 0 1 1 1
  line L1512 (-11.9913, 30.3398) -> (-11.9786, 30.2932) construction
  line L1513 (-11.9786, 30.2932) -> (-11.9786, 30.2467) construction
  spline S388 degree 2 poles (-11.9786, 30.2467) (-11.9786, 30.0054) (-12.241, 30.0054) knots 0 0 0 1 1 1
  line L1514 (-11.9786, 30.2467) -> (-11.9786, 30.0054) construction
  line L1515 (-11.9786, 30.0054) -> (-12.241, 30.0054) construction
  spline S389 degree 2 poles (-12.241, 30.0054) (-12.4146, 30.0054) (-12.4696, 30.179) knots 0 0 0 1 1 1
  line L1516 (-12.241, 30.0054) -> (-12.4146, 30.0054) construction
  line L1517 (-12.4146, 30.0054) -> (-12.4696, 30.179) construction
  spline S390 degree 2 poles (-18.0947, 30.5091) (-17.6757, 30.5091) (-17.0831, 31.1017) (-17.0831, 31.5207) knots 0 0 0 1 2 2 2
  line L1518 (-18.0947, 30.5091) -> (-17.6757, 30.5091) construction
  line L1519 (-17.6757, 30.5091) -> (-17.0831, 31.1017) construction
  line L1520 (-17.0831, 31.1017) -> (-17.0831, 31.5207) construction
  spline S391 degree 2 poles (-17.0831, 31.5207) (-17.0831, 31.9397) (-17.6757, 32.5323) (-18.0947, 32.5323) knots 0 0 0 1 2 2 2
  line L1521 (-17.0831, 31.5207) -> (-17.0831, 31.9397) construction
  line L1522 (-17.0831, 31.9397) -> (-17.6757, 32.5323) construction
  line L1523 (-17.6757, 32.5323) -> (-18.0947, 32.5323) construction
  line L1524 (-18.0947, 30.0012) -> (-19.3602, 30.0012)
  spline S392 degree 2 poles (-19.3602, 30.0012) (-19.4618, 30.0012) (-19.6142, 30.1536) (-19.6142, 30.2551) knots 0 0 0 1 2 2 2
  line L1525 (-19.3602, 30.0012) -> (-19.4618, 30.0012) construction
  line L1526 (-19.4618, 30.0012) -> (-19.6142, 30.1536) construction
  line L1527 (-19.6142, 30.1536) -> (-19.6142, 30.2551) construction
  line L1528 (-19.6142, 30.2551) -> (-19.6142, 34.8136)
  spline S393 degree 2 poles (-19.6142, 34.8136) (-19.6142, 34.9152) (-19.4618, 35.0676) (-19.3602, 35.0676) knots 0 0 0 1 2 2 2
  line L1529 (-19.6142, 34.8136) -> (-19.6142, 34.9152) construction
  line L1530 (-19.6142, 34.9152) -> (-19.4618, 35.0676) construction
  line L1531 (-19.4618, 35.0676) -> (-19.3602, 35.0676) construction
  line L1532 (-19.3602, 35.0676) -> (-17.0831, 35.0676)
  spline S394 degree 2 poles (-17.0831, 35.0676) (-16.8291, 35.0676) (-16.8291, 34.8136) knots 0 0 0 1 1 1
  line L1533 (-17.0831, 35.0676) -> (-16.8291, 35.0676) construction
  line L1534 (-16.8291, 35.0676) -> (-16.8291, 34.8136) construction
  spline S395 degree 2 poles (-16.8291, 34.8136) (-16.8291, 34.5597) (-17.0831, 34.5597) knots 0 0 0 1 1 1
  line L1535 (-16.8291, 34.8136) -> (-16.8291, 34.5597) construction
  line L1536 (-16.8291, 34.5597) -> (-17.0831, 34.5597) construction
  spline S396 degree 2 poles (-18.0947, 33.0402) (-17.464, 33.0402) (-16.5752, 32.1471) (-16.5752, 31.5207) knots 0 0 0 1 2 2 2
  line L1537 (-18.0947, 33.0402) -> (-17.464, 33.0402) construction
  line L1538 (-17.464, 33.0402) -> (-16.5752, 32.1471) construction
  line L1539 (-16.5752, 32.1471) -> (-16.5752, 31.5207) construction
  spline S397 degree 2 poles (-16.5752, 31.5207) (-16.5752, 30.8943) (-17.4683, 30.0012) (-18.0947, 30.0012) knots 0 0 0 1 2 2 2
  line L1540 (-16.5752, 31.5207) -> (-16.5752, 30.8943) construction
  line L1541 (-16.5752, 30.8943) -> (-17.4683, 30.0012) construction
  line L1542 (-17.4683, 30.0012) -> (-18.0947, 30.0012) construction
  spline S398 degree 2 poles (12.9798, 88.4511) (12.9703, 88.125) (12.9467, 87.5246) (12.9325, 87.2835) knots 0 0 0 1 2 2 2
  line L1543 (12.9798, 88.4511) -> (12.9703, 88.125) construction
  line L1544 (12.9703, 88.125) -> (12.9467, 87.5246) construction
  line L1545 (12.9467, 87.5246) -> (12.9325, 87.2835) construction
  spline S399 degree 2 poles (12.9325, 87.2835) (12.9088, 86.669) (12.7954, 85.837) (12.7103, 85.5865) knots 0 0 0 1 2 2 2
  line L1546 (12.9325, 87.2835) -> (12.9088, 86.669) construction
  line L1547 (12.9088, 86.669) -> (12.7954, 85.837) construction
  line L1548 (12.7954, 85.837) -> (12.7103, 85.5865) construction
  spline S400 degree 2 poles (12.7103, 85.5865) (12.6252, 85.3265) (12.4172, 85.0381) (12.2849, 84.9199) knots 0 0 0 1 2 2 2
  line L1549 (12.7103, 85.5865) -> (12.6252, 85.3265) construction
  line L1550 (12.6252, 85.3265) -> (12.4172, 85.0381) construction
  line L1551 (12.4172, 85.0381) -> (12.2849, 84.9199) construction
  spline S401 degree 2 poles (12.2849, 84.9199) (12.1525, 84.8017) (11.85, 84.6836) (11.6561, 84.6836) knots 0 0 0 1 2 2 2
  line L1552 (12.2849, 84.9199) -> (12.1525, 84.8017) construction
  line L1553 (12.1525, 84.8017) -> (11.85, 84.6836) construction
  line L1554 (11.85, 84.6836) -> (11.6561, 84.6836) construction
  spline S402 degree 2 poles (11.6561, 84.6836) (11.5947, 84.6836) (11.3961, 84.693) (11.3583, 84.693) knots 0 0 0 1 2 2 2
  line L1555 (11.6561, 84.6836) -> (11.5947, 84.6836) construction
  line L1556 (11.5947, 84.6836) -> (11.3961, 84.693) construction
  line L1557 (11.3961, 84.693) -> (11.3583, 84.693) construction
  spline S403 degree 2 poles (11.3961, 85.3359) (11.4245, 85.3359) (11.486, 85.3265) (11.5238, 85.3265) knots 0 0 0 1 2 2 2
  line L1558 (11.3961, 85.3359) -> (11.4245, 85.3359) construction
  line L1559 (11.4245, 85.3359) -> (11.486, 85.3265) construction
  line L1560 (11.486, 85.3265) -> (11.5238, 85.3265) construction
  spline S404 degree 2 poles (11.5238, 85.3265) (11.6183, 85.3265) (11.798, 85.3832) (11.8689, 85.4541) knots 0 0 0 1 2 2 2
  line L1561 (11.5238, 85.3265) -> (11.6183, 85.3265) construction
  line L1562 (11.6183, 85.3265) -> (11.798, 85.3832) construction
  line L1563 (11.798, 85.3832) -> (11.8689, 85.4541) construction
  spline S405 degree 2 poles (11.8689, 85.4541) (12.0627, 85.6479) (12.2423, 86.6075) (12.2801, 87.4726) knots 0 0 0 1 2 2 2
  line L1564 (11.8689, 85.4541) -> (12.0627, 85.6479) construction
  line L1565 (12.0627, 85.6479) -> (12.2423, 86.6075) construction
  line L1566 (12.2423, 86.6075) -> (12.2801, 87.4726) construction
  spline S406 degree 2 poles (12.2801, 87.4726) (12.299, 87.794) (12.3274, 88.6686) (12.3369, 89.0704) knots 0 0 0 1 2 2 2